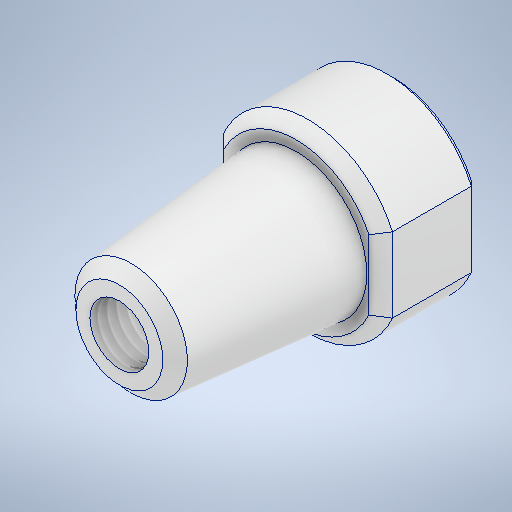
# Autodesk Inventor part: Linear Actuator Plate Holder
Saved by Autodesk Inventor 2025.3 (Build 293356000, 356)
## iProperties
Created: 2025-10-10
Part Number: Linear Actuator Plate Holder
Material: Aluminum 6061
Document SubType Name: Modeling
Designer: Haggag
Density: 2.7 g/cm^3
Appearance: Aluminum - Flat
Author: Haggag
Autodesk Inventor part; units mm, degrees
ref_plane "YZ Plane" through (0, 0, 0) normal (1, 0, 0) x (0, 1, 0)
ref_plane "XZ Plane" through (0, 0, 0) normal (0, 1, 0) x (-1, 0, 0)
ref_plane "XY Plane" through (0, 0, 0) normal (0, 0, 1) x (1, 0, 0)
sketch "Sketch1" plane through (0, 0, 0) normal (0, 0, 1) x (1, 0, 0)
  line L0 (7.1859, 2.9745) -> (7.1859, -3.1752)
  line L1 (0, 6) -> (0, -6)
  line L2 (-7.1859, 2.9745) -> (-7.1859, -3.1752)
  arc A0 (-7.1859, -3.1752) -> (7.1859, -3.1752) centre (0, 0) ccw
  circle A1 centre (0, 0) radius 4.5
  line L3 (0, 0) -> (-2.4413, 0)
  arc A2 (7.1859, 3.1752) -> (-7.1859, 3.1752) centre (0, 0) ccw
  line L4 (-7.1859, 3.1752) -> (-7.1859, 2.8831)
  line L5 (7.1859, 3.1752) -> (7.1859, 2.9745)
  dimension "d27" = 9
  constraints: 12 end point, 4 point on circle, 4 symmetric about line, 3 centre point, 3 vertical, 1 coincident, 1 horizontal, 1 point on line, 1 other
  measures "d27" diameter of A1
extrude "Extrusion1" add sketch "Sketch1" along normal blind 6.2 contours L0 A0 L2 L4 A2 L5 | A1 L1 | L1 A1
sketch "Sketch3" plane through (0, 0, 6.2) normal (0, 0, 1) x (-1, 0, 0)
  circle A0 centre (0, 0) radius 6
  dimension "d21" = 12
  constraints: 1 centre point, 1 coincident
  measures "d21" diameter of A0
extrude "Extrusion3" add sketch "Sketch3" along normal blind 15 draft -5
chamfer "Chamfer1" distance 1 angle 45 1 edges at (4.6877, 0, 21.2)
chamfer "Chamfer2" distance 1 angle 45 4 edges at (0, -7.8562, 6.2) (7.1859, 0, 6.2) (-7.1859, 0, 6.2) (0, 7.8562, 6.2)
sketch "Sketch4" plane through (0, 0, 21.2) normal (0, 0, 1) x (1, 0, 0)
  circle A0 centre (0, 0) radius 2.5
  dimension "d16" = 5
  constraints: 1 centre point, 1 coincident
  measures "d16" diameter of A0
extrude "Extrusion4" cut sketch "Sketch4" against normal blind 12
thread "Thread1" size "M5x0.8" class "6H" standard "ANSI Metric M Profile" full length
extrude "Extrusion7" cut sketch "Sketch1" along normal blind 7.3 contours A1 L1 | L1 A1
extrude "Extrusion8" add sketch "Sketch1" against normal blind 2
chamfer "Chamfer4" distance 0.5 angle 45 4 edges at (0, -7.8562, -2) (-7.1859, 0, -2) (0, 7.8562, -2) (7.1859, 0, -2)
body "Solid1"
